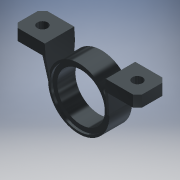
# Autodesk Inventor part: lagerblock
Saved by Autodesk Inventor 2017 (Build 210142000, 142)
## iProperties
Part Number: lagerblock
Material: Gusseisen, grau, ASTM A48 Klasse 20
Document SubType Name: Modeling
Designer: Till
Density: 7.3953 g/cm^3
Appearance: Eisen - grau
Author: Till
Autodesk Inventor part; units mm, degrees
ref_plane "YZ Plane" through (0, 0, 0) normal (1, 0, 0) x (0, 1, 0)
ref_plane "XZ Plane" through (0, 0, 0) normal (0, 1, 0) x (-1, 0, 0)
ref_plane "XY Plane" through (0, 0, 0) normal (0, 0, 1) x (1, 0, 0)
sketch "Skizze1" plane through (0, 0, 0) normal (0, 0, 1) x (1, 0, 0)
  line L0 (0, 0) -> (-2, 0)
  line L1 (-2, 0) -> (-2, -1)
  line L2 (-2, -1) -> (-3, -1)
  line L3 (-3, -1) -> (-3, 9)
  line L4 (-3, 9) -> (-2, 9)
  line L5 (-2, 9) -> (-2, 8)
  line L6 (-2, 8) -> (0, 8)
  line L7 (0, 8) -> (0, 0)
  line L8 (10.5, 10.652115) -> (10.5, -3.008314) construction
  dimension "d0" = 3
  dimension "d1" = 10
  dimension "d2" = 8
  dimension "d3" = 1
  dimension "d4" = 2
  dimension "d5" = 10.5
  constraints: 18 end point, 6 perpendicular, 2 point on line, 1 horizontal, 1 vertical
  measures "d0" distance between parallel lines of L7 L3
  measures "d1" distance between parallel lines of L2 L4
  measures "d2" distance between parallel lines of L0 L6
  measures "d3" distance between parallel lines of L6 L4
  measures "d4" distance between parallel lines of L5 L7
  measures "d5" distance between parallel lines of L8 L7
sketch "Skizze1 outline for Umdrehung1" plane through (0, 0, 0) normal (0, 0, 1) x (1, 0, 0)
  line L0 (0, 0) -> (-2, 0)
  line L1 (-2, 0) -> (-2, -1)
  line L2 (-2, -1) -> (-3, -1)
  line L3 (-3, -1) -> (-3, 9)
  line L4 (-3, 9) -> (-2, 9)
  line L5 (-2, 9) -> (-2, 8)
  line L6 (-2, 8) -> (0, 8)
  line L7 (0, 8) -> (0, 0)
revolve "Umdrehung1" add sketch "Skizze1 outline for Umdrehung1" angle 360 about axis through (10.5, 10.652115, 0) along (0, -1, 0)
sketch "Skizze2" plane through (10.5, -1, 0) normal (0, -1, 0) x (1, 0, 0)
  circle A0 centre (0, 0) radius 13.5 construction
  line L0 (-13.499999, -0.004969) -> (1.488599, -0.004969) construction
  line L1 (-13.5, 14.995031) -> (-27.5, 14.995031)
  line L2 (-27.5, 14.995031) -> (-27.5, 9.995031)
  circle A1 centre (0, 0) radius 12.5 construction
  circle A2 centre (0, 0) radius 13.5
  circle A3 centre (0, 0) radius 12.5
  circle A4 centre (0, 0) radius 12.5
  line L3 (-27.5, 9.995031) -> (-14.5, 9.995031)
  line L4 (-14.5, 9.995031) -> (-13.499999, -0.004969)
  line L5 (-0.042524, -33.95519) -> (-0.042524, 19.973998) construction
  line L6 (13.414952, 14.995031) -> (27.414952, 14.995031)
  line L7 (27.414952, 14.995031) -> (27.414952, 9.995031)
  line L8 (12.499991, -0.004969) -> (13.414952, 14.995031)
  line L9 (27.414952, 9.995031) -> (14.414952, 9.995031)
  line L10 (14.414952, 9.995031) -> (13.414951, -0.004969)
  line L11 (-13.5, 14.995031) -> (-12.499999, -0.004969)
  circle A5 centre (0, 0) radius 12.5
  line L12 (-12.499999, -0.004969) -> (-13.499999, -0.004969)
  line L13 (13.414951, -0.004969) -> (12.499991, -0.004969)
  point P0 (-10.5, 0)
  point P1 (10.414952, 0)
  dimension "d9" = 15
  dimension "d11" = 5
  dimension "d12" = 13
  dimension "d13" = 14
  dimension "d14" = 27.5
  constraints: 28 end point, 6 symmetric about line, 3 horizontal, 2 collinear, 1 perpendicular, 1 vertical, 6 other
  measures "d9" distance of L0.start L1.start
  measures "d11" distance of L1.end L2.end
  measures "d12" distance of L2.end L3.end
  measures "d13" distance from line of L2 L1.start
  measures "d14" distance from line of point (0, 0) L2
sketch "Skizze2 outline for Extrusion1" plane through (10.5, -1, 0) normal (0, -1, 0) x (1, 0, 0)
  line L0 (12.499991, -0.004969) -> (13.414951, -0.004969)
  line L1 (13.414952, 14.995031) -> (12.499991, -0.004969)
  line L2 (27.414952, 14.995031) -> (13.414952, 14.995031)
  line L3 (27.414952, 9.995031) -> (27.414952, 14.995031)
  line L4 (14.414952, 9.995031) -> (27.414952, 9.995031)
  line L5 (13.414951, -0.004969) -> (14.414952, 9.995031)
  line L6 (-13.499999, -0.004969) -> (-14.5, 9.995031)
  line L7 (-14.5, 9.995031) -> (-27.5, 9.995031)
  line L8 (-27.5, 9.995031) -> (-27.5, 14.995031)
  line L9 (-27.5, 14.995031) -> (-13.5, 14.995031)
  line L10 (-13.5, 14.995031) -> (-12.499999, -0.004969)
  line L11 (-12.499999, -0.004969) -> (-13.499999, -0.004969)
extrude "Extrusion1" add sketch "Skizze2 outline for Extrusion1" against normal blind 11.5 and the other way blind 1.5
sketch "Skizze5" plane through (-17, -2.5, 14.995031) normal (-1, 0, 0) x (0, 0, 1)
  line L0 (-15, 13) -> (-15, 11.5) projected
  line L1 (-5, 13) -> (-5, 0) projected
  line L2 (-15, 11.5) -> (-5, 13)
  line L3 (-5, 13) -> (-15, 13)
  line L4 (-15, 13) -> (-15, 11.5)
  line L5 (-15, 1.5) -> (-15, 11.5) projected
  line L6 (-15, 1.5) -> (-5, 0)
  line L7 (0, 0) -> (-15, 0) projected
  line L8 (-15, 1.5) -> (-15, 0) projected
  line L9 (-15, 0) -> (-15, 1.5)
  line L10 (-15, 0) -> (-5, 0)
  point P0 (-14.995031, 2.5)
  constraints: 12 end point, 2 collinear, 2 perpendicular, 2 point on line
sketch "Skizze5 outline for Extrusion4" plane through (-17, -2.5, 14.995031) normal (-1, 0, 0) x (0, 0, 1)
  line L0 (-15, 13) -> (-15, 11.5)
  line L1 (-5, 13) -> (-15, 13)
  line L2 (-15, 11.5) -> (-5, 13)
  line L3 (-5, 0) -> (-15, 1.5)
  line L4 (-15, 0) -> (-5, 0)
  line L5 (-15, 1.5) -> (-15, 0)
extrude "Extrusion4" cut sketch "Skizze5 outline for Extrusion4" against normal through all
chamfer "Fase1" distance 2 angle 45 4 edges at (-17, -2.5, 12.495) (-17, 10.5, 12.495) (37.915, -2.5, 12.495) (37.915, 10.5, 12.495)
hole "Bohrung1" at (31.414952, 4, 9.995031) direction (0, 0, 1) diameter 4.5 end through all
hole "Bohrung2" at (-10.5, 4, 9.995031) direction (0, 0, 1) diameter 4.5 end through all
